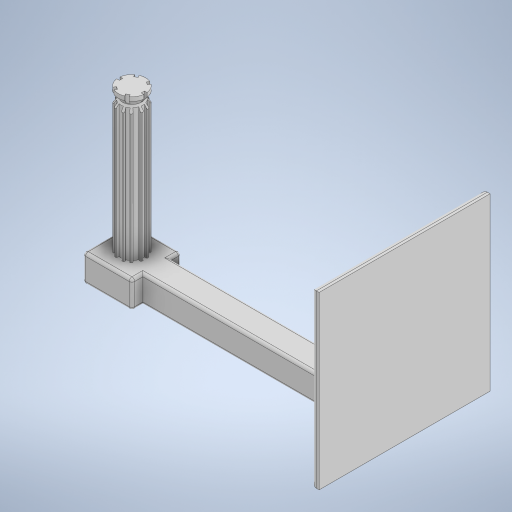
# Autodesk Inventor part: StandV1
Saved by Autodesk Inventor 2024 (Build 280153000, 153)
## iProperties
Created: 2024-01-02
Part Number: StandV1
Material: Generisch
Document SubType Name: Modeling
Designer: chris
Density: 1 g/cm^3
Appearance: Vorgabe
Author: chris
Autodesk Inventor part; units mm, degrees
ref_plane "YZ Plane" through (0, 0, 0) normal (1, 0, 0) x (0, 1, 0)
ref_plane "XZ Plane" through (0, 0, 0) normal (0, 1, 0) x (-1, 0, 0)
ref_plane "XY Plane" through (0, 0, 0) normal (0, 0, 1) x (1, 0, 0)
sketch "Skizze1" plane through (0, 0, 0) normal (0, 0, 1) x (1, 0, 0)
  circle A0 centre (0, 0) radius 5
  dimension "d0" = 10
  constraints: 1 centre point, 1 coincident
  measures "d0" diameter of A0
extrude "Extrusion1" add sketch "Skizze1" along normal mid plane 62.7
sketch "Skizze2" plane through (0, 0, -31.35) normal (0, 0, -1) x (-1, 0, 0)
  point P0 (0, 0)
sketch "Skizze3" plane through (0, 0, 0) normal (1, 0, 0) x (0, 1, 0)
  line L0 (-5, -31.35) -> (5, -31.35) projected
  line L1 (5, -31.35) -> (5, 31.35) projected
  line L2 (-5, -31.35) -> (5, -31.35)
  line L3 (5, -31.35) -> (5, -21.35)
  line L4 (5, -21.35) -> (-5, -21.35)
  line L5 (-5, -21.35) -> (-5, -31.35)
  point P0 (0, 0)
  dimension "d3" = 10
  constraints: 8 end point, 2 parallel, 1 horizontal, 1 perpendicular, 1 point on line
  measures "d3" distance of L3.end L2.end
extrude "Extrusion2" add sketch "Skizze3" along normal blind 100
sketch "Skizze4" plane through (0, -5, -21.35) normal (0, 0, 1) x (1, 0, 0)
  line L0 (100, 10) -> (100, 0) projected
  line L1 (0, 10) -> (100, 10) projected
  line L2 (100, 0) -> (97, 0)
  line L3 (97, 0) -> (97, 10)
  line L4 (97, 10) -> (100, 10)
  line L5 (100, 10) -> (100, 0)
  point P0 (0, 5)
  dimension "d6" = 3
  constraints: 8 end point, 2 parallel, 1 horizontal, 1 perpendicular, 1 point on line
  measures "d6" distance of L3.end L4.end
extrude "Extrusion3" add sketch "Skizze4" along normal blind 51.2
chamfer "Fasen1" distance 10 angle 45 1 edges at (97, 0, -21.35)
sketch "Skizze5" plane through (97, -5, 29.85) normal (-1, 0, 0) x (0, 0, 1)
  line L0 (-41.2, 0) -> (0, 0) construction
  line L1 (0, 0) -> (-61.2, 10) construction
  line L2 (-61.2, 0) -> (0, 0) construction
  line L3 (-61.2, 10) -> (-61.2, 0) construction
  line L4 (0, 10) -> (-61.2, 0) construction
  line L5 (1.5, 36.35) -> (-61.2, 36.35)
  line L6 (-61.2, 36.35) -> (-61.2, -26.35)
  line L7 (-61.2, -26.35) -> (1.5, -26.35)
  line L8 (1.5, -26.35) -> (1.5, 36.35)
  line L9 (1.5, 36.35) -> (-61.2, -26.35) construction
  line L10 (-61.2, 36.35) -> (1.5, -26.35) construction
  point P0 (-29.85, 5)
  dimension "d12" = 62.7
  dimension "d30" = 62.7
  constraints: 16 end point, 2 midpoint, 2 parallel, 1 horizontal, 1 perpendicular
  measures "d12" distance of L6.end L5.end
  measures "d30" distance of L6.end L7.end
extrude "Extrusion4" add sketch "Skizze5" against normal blind 3
chamfer "Fasen2" distance 4 angle 45 2 edges at (97, 5, -21.35) (97, -5, -21.35)
fillet "Rundung1" radius 2 5 edges at (97, 31.35, 0) (97, 0, 31.35) (97, -31.35, 0) (97, -20.175, -31.35) (97, 20.175, -31.35)
fillet "Rundung2" radius 1 9 edges at (43.5, -5, -21.35) (43.5, 5, -21.35) (-5, 0, -31.35) (46.5, 5, -31.35) (46.5, -5, -31.35) (98, 10, -31.35) (95, 7, -31.35) (98, -10, -31.35) (95, -7, -31.35)
sketch "Skizze6" plane through (0, 0, 0) normal (0, 1, 0) x (-1, 0, 0)
  line L0 (5, -30.35) -> (5, 31.35) projected
  line L1 (5, 27.85) -> (3.5, 27.85) construction
  line L2 (5, 31.35) -> (-5, 31.35) projected
  line L3 (3.5, 27.85) -> (5, 25.85)
  line L4 (3.5, 27.85) -> (5, 29.85)
  line L5 (5, 25.85) -> (5, 29.85)
  line L6 (0, -42.84) -> (0, 42.84) projected
  point P0 (0, 0)
  dimension "d20" = 1.5
  dimension "d21" = 3.5
  dimension "d22" = 2
  dimension "d23" = 2
  constraints: 8 end point, 3 point on line, 1 collinear, 1 horizontal
  measures "d20" distance of L1.start L1.end
  measures "d21" distance between parallel lines of L2 L1
  measures "d22" distance from line of L1 L3.end
  measures "d23" distance from line of L1 L4.end
revolve "Umdrehung1" cut sketch "Skizze6" angle 360 about axis through (0, 0, -10) along (0, 0, 1)
sketch "Skizze7" plane through (3, 4, -21.35) normal (0, 0, 1) x (1, 0, 0)
  circle A0 centre (-3, -4) radius 5 construction
  line L0 (2, -4) -> (2, -9) construction
  line L1 (2, -9) -> (-8, 1) construction
  line L2 (6, 5) -> (-12, 5)
  line L3 (-12, 5) -> (-12, -13)
  line L4 (-12, -13) -> (6, -13)
  line L5 (6, -13) -> (6, 5)
  line L6 (6, 5) -> (-12, -13) construction
  line L7 (-12, 5) -> (6, -13) construction
  dimension "d26" = 4
  dimension "d27" = 4
  constraints: 16 end point, 2 midpoint, 2 parallel, 2 vertical, 1 horizontal, 1 horizontal alignment, 1 perpendicular, 1 other
extrude "Extrusion5" add sketch "Skizze7" against normal blind 10
fillet "Rundung3" radius 1 14 edges at (-9, -9, -26.35) (9, -9, -26.35) (0, -9, -21.35) (-9, 0, -21.35) (0, 9, -21.35) (9, 6.5, -21.35) (9, -6.5, -21.35) (9, 9, -26.35) (0, 9, -31.35) (-9, 9, -26.35) (-9, 0, -31.35) (0, -9, -31.35) (9, -6.5, -31.35) (9, 6.5, -31.35)
sketch "Skizze8" plane through (0, 0, 0) normal (0, 0, 1) x (1, 0, 0)
  circle A0 centre (0, 0) radius 5 projected
  line L0 (-5, 0) -> (-4, 0) construction
  line L1 (-4, 0) -> (-4, 0.6)
  line L2 (-4, 0) -> (-4, -0.6)
  line L3 (-4, -0.6) -> (-4.9639, -0.6)
  line L4 (-4, 0.6) -> (-4.9639, 0.6)
  dimension "d32" = 1
  dimension "d33" = 0.6
  dimension "d34" = 0.6
  constraints: 10 end point, 3 point on circle, 2 horizontal, 1 parallel, 1 perpendicular, 1 vertical
  measures "d32" distance of L0.start L0.end
  measures "d33" distance of L0.end L1.end
  measures "d34" distance of L0.end L2.end
extrude "Extrusion6" cut sketch "Skizze8" along normal blind 40 and the other way blind 21.35 contours L4 L1 L2 L3 A0 picked at (-4.332, -0.2668)
pattern_circular "Runde Anordnung1" count 6 over 360 about axis through (0, 0, -10) along (0, 0, 1) of "Extrusion6"
sketch "Skizze9" plane through (0, 0, 0) normal (0, 0, 1) x (1, 0, 0)
  circle A0 centre (0, 0) radius 4
  arc A1 (-3.0015, 3.9988) -> (-4.9639, 0.6) centre (0, 0) ccw projected
  line L0 (-2.5196, 3.1641) -> (-3.0015, 3.9988) projected
  line L1 (-3.7542, 3.3024) -> (-3.0033, 2.642)
  line L2 (-4.9639, 0.6) -> (-4, 0.6) projected
  line L3 (-4.7371, 1.6) -> (-3.7897, 1.28)
  point P0 (-3.8991, -0.8927)
  point P1 (-4.43, 0.6)
  point P2 (-2.7346, 3.5365)
  dimension "d42" = 1
  dimension "d51" = 1
  dimension "d53" = 8
  constraints: 5 point on circle, 4 end point, 2 line through centre, 1 centre point, 1 coincident
  measures "d42" distance from line of L1.start L0
  measures "d51" distance from line of L2 L3.start
  measures "d53" diameter of A0
extrude "Extrusion7" cut sketch "Skizze9" along normal blind 28 and the other way blind 21.35 contours A0 L3 A1 L1
pattern_circular "Runde Anordnung2" count 6 over 360 about axis through (0, 0, -10) along (0, 0, 1) of "Extrusion7"
fillet "Rundung4" radius 0.29 18 edges at (-0.9829, -4.9024, 2.25) (-1.9623, -4.5988, 2.25) (-3.0015, -3.9988, 2.25) (-4.7371, -1.6, 2.25) (-4.9639, -0.6, 2.25) (-4.9639, 0.6, 2.25) (-3.7542, 3.3024, 2.25) (-3.0015, 3.9988, 2.25) (-1.9623, 4.5988, 2.25) (0.9829, 4.9024, 2.25) (1.9623, 4.5988, 2.25) (3.0015, 3.9988, 2.25) (4.7371, 1.6, 2.25) (4.9639, 0.6, 2.25) (4.9639, -0.6, 2.25) (1.9623, -4.5988, 2.25) (3.0015, -3.9988, 2.25) (3.7542, -3.3024, 2.25)
fillet "Rundung5" radius 0.29 6 edges at (-4.7371, 1.6, 2.25) (-0.9829, 4.9024, 2.25) (3.7542, 3.3024, 2.25) (4.7371, -1.6, 2.25) (0.9829, -4.9024, 2.25) (-3.7542, -3.3024, 2.25)
